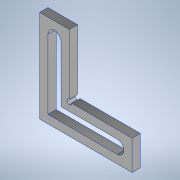
# Autodesk Inventor part: Kabelhalterung_V1
Saved by Autodesk Inventor 2022 (Build 260153000, 153)
## iProperties
Created: 2022-04-11
Part Number: Kabelhalterung_V1
Material: Generic
Document SubType Name: Modeling
Designer: richa
Density: 1 g/cm^3
Appearance: Aluminum - Flat
Author: richa
Autodesk Inventor part; units mm, degrees
ref_plane "YZ Plane" through (0, 0, 0) normal (1, 0, 0) x (0, 1, 0)
ref_plane "XZ Plane" through (0, 0, 0) normal (0, 1, 0) x (-1, 0, 0)
ref_plane "XY Plane" through (0, 0, 0) normal (0, 0, 1) x (1, 0, 0)
sketch "Sketch1" plane through (0, 0, 0) normal (0, 0, 1) x (1, 0, 0)
  line L0 (0, 0) -> (0, 50)
  line L1 (0, 50) -> (12, 50)
  line L2 (12, 50) -> (12, 12)
  line L3 (12, 12) -> (50, 12)
  line L4 (50, 12) -> (50, 0)
  line L5 (50, 0) -> (0, 0)
  dimension "d0" = 50
  dimension "d1" = 12
  dimension "d2" = 38
  dimension "d3" = 38
  constraints: 12 end point, 5 perpendicular, 1 vertical
  measures "d0" distance of L0.start L0.end
  measures "d1" distance of L0.end L1.end
  measures "d2" distance of L1.end L2.end
  measures "d3" distance of L2.end L3.end
extrude "Extrusion1" add sketch "Sketch1" along normal blind 5
sketch "Sketch2" plane through (0, 0, 5) normal (0, 0, 1) x (1, 0, 0)
  line L0 (10, 44) -> (10, 2)
  line L1 (10, 2) -> (2, 2)
  line L2 (2, 2) -> (2, 44)
  line L3 (12, 12) -> (12, 50) projected
  line L4 (12, 50) -> (0, 50) projected
  arc A0 (10, 44) -> (2, 44) centre (6, 44) ccw
  line L5 (0, 0) -> (50, 0) projected
  line L6 (2, 2) -> (44, 2)
  line L7 (44, 10) -> (2, 10)
  line L8 (2, 10) -> (2, 2)
  arc A1 (44, 2) -> (44, 10) centre (44, 6) ccw
  line L9 (50, 0) -> (50, 12) projected
  line L10 (50, 12) -> (12, 12) projected
  point P0 (10, 2)
  point P1 (10, 10)
  dimension "d6" = 8
  dimension "d7" = 2
  dimension "d9" = 4
  dimension "d10" = 6
  dimension "d11" = 2
  dimension "d12" = 8
  dimension "d13" = 6
  dimension "d14" = 2
  dimension "d15" = 4
  constraints: 12 end point, 4 point on circle, 2 centre point, 2 parallel, 1 horizontal
  measures "d6" distance of L0.end L1.end
  measures "d7" distance between parallel lines of L3 L0
  measures "d9" radius of A0
  measures "d10" distance from line of A0.centre L4
  measures "d11" distance between parallel lines of L5 L1
  measures "d12" distance of L7.start L6.end
  measures "d13" distance from line of L9 A1.centre
  measures "d14" distance between parallel lines of L7 L10
  measures "d15" radius of A1
extrude "Extrusion2" cut sketch "Sketch2" against normal through all
sketch "Sketch3" plane through (0, 0, 5) normal (0, 0, 1) x (1, 0, 0)
  line L0 (15, 15) -> (15, 50)
  line L1 (-3, 50) -> (-3, 0)
  line L2 (15, 15) -> (53, 15)
  line L3 (50, -3) -> (-3, -3)
  line L4 (-3, -3) -> (-3, 16.0843)
  line L5 (0, 50) -> (0, 0) projected
  line L6 (12, 12) -> (12, 50) projected
  line L7 (50, 12) -> (12, 12) projected
  line L8 (0, 0) -> (50, 0) projected
  line L9 (15, 50) -> (15, 53)
  line L10 (15, 53) -> (-3, 53)
  line L11 (-3, 53) -> (-3, 50)
  line L12 (50, -3) -> (53, -3)
  line L13 (53, -3) -> (53, 15)
  line L14 (12, 50) -> (0, 50) projected
  line L15 (50, 0) -> (50, 12) projected
  dimension "d18" = 3
  dimension "d19" = 3
  dimension "d20" = 3
  dimension "d21" = 3
  dimension "d24" = 3
  dimension "d25" = 3
  constraints: 20 end point, 3 parallel, 2 horizontal, 1 collinear, 1 perpendicular, 1 point on line
  measures "d18" distance between parallel lines of L5 L1
  measures "d19" distance between parallel lines of L6 L0
  measures "d20" distance between parallel lines of L7 L2
  measures "d21" distance between parallel lines of L8 L3
  measures "d24" distance between parallel lines of L15 L13
  measures "d25" distance between parallel lines of L14 L10
extrude "Extrusion3" add sketch "Sketch3" against normal blind 5
sketch "Sketch4" plane through (0, 0, 5) normal (0, 0, 1) x (1, 0, 0)
  line L0 (53, 15) -> (15, 15) projected
  circle A0 centre (15, 15) radius 1.5
  point P0 (0, 0)
  dimension "d28" = 3
  constraints: 1 centre point
  measures "d28" diameter of A0
extrude "Extrusion4" cut sketch "Sketch4" against normal blind 5
body "Solid1"
